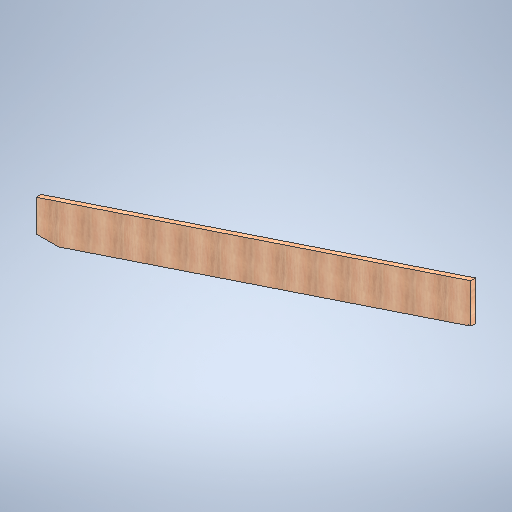
# Autodesk Inventor part: Rafter
Saved by Autodesk Inventor 2025 (Build 290162010, 162A)
## iProperties
Created: 2024-09-15
Part Number: Rafter
Material: Wood (Birch)
Document SubType Name: Modeling
Designer: Tom
Density: 0.55 g/cm^3
Appearance: Birch - Natural Polished
Author: Tom
Autodesk Inventor part; units mm, degrees
ref_plane "YZ Plane" through (0, 0, 0) normal (1, 0, 0) x (0, 1, 0)
ref_plane "XZ Plane" through (0, 0, 0) normal (0, 1, 0) x (-1, 0, 0)
ref_plane "XY Plane" through (0, 0, 0) normal (0, 0, 1) x (1, 0, 0)
sketch "Sketch1" plane through (0, 0, 0) normal (0, 0, 1) x (1, 0, 0)
  line L0 (0, 0) -> (3230.5625, 1077.3862)
  line L1 (3230.5625, 1385.3019) -> (-174.625, 249.6786)
  line L2 (0, 0) -> (-174.625, 0)
  line L3 (-174.625, 0) -> (-174.625, 249.6786)
  line L4 (-174.625, 249.6786) -> (1499.203, 807.8969)
  line L5 (3230.5625, 1077.3862) -> (3213.1, 1077.3862)
  line L6 (3230.5625, 1077.3862) -> (3230.5625, 1385.3019)
  line L7 (-139.7, 0) -> (-139.7, 261.326)
  line L8 (3213.1, 1071.5625) -> (3213.1, 1379.4782)
  line L9 (-174.625, 249.6786) -> (-91.3577, 0)
  dimension "d5" = 292.1
  dimension "d17" = 139.7
  dimension "d19" = 3352.8
  dimension "d23" = 17.4625
  dimension "d27" = 1071.5625
  dimension "d28" = 34.925
  constraints: 20 end point, 6 point on line, 4 vertical, 2 coincident, 2 horizontal, 1 collinear, 1 perpendicular
  measures "d5" distance between parallel lines of L1 L0
  measures "d17" distance from line of L7 point (0, 0)
  measures "d19" distance between parallel lines of L7 L8
  measures "d23" distance between parallel lines of L6 L8
  measures "d27" vertical distance of L8.start point (0, 0)
  measures "d28" distance between parallel lines of L3 L7
extrude "Extrusion1" add sketch "Sketch1" along normal blind 38.1 contours L2 L9 L7 L1 L8 L0 | L2 L7 L9 | L5 L8 L1 L6 | L2 L3 L9 L7 | L9 L1 L7
ref_plane "Work Plane1" through (-174.625, 249.6786, 0) normal (-0.9486364, -0.3163684, 0) x (0.3163684, -0.9486364, 0)
body "Solid1"
